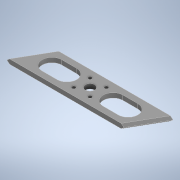
# Autodesk Inventor part: rotorV2
Saved by Autodesk Inventor 2021 (Build 250183000, 183)
## iProperties
Created: 2022-10-22
Part Number: rotorV2
Material: Generic
Document SubType Name: Modeling
Designer: ermoz
Density: 1 g/cm^3
Appearance: Default
Author: ermoz
Autodesk Inventor part; units mm, degrees
ref_plane "YZ Plane" through (0, 0, 0) normal (1, 0, 0) x (0, 1, 0)
ref_plane "XZ Plane" through (0, 0, 0) normal (0, 1, 0) x (-1, 0, 0)
ref_plane "XY Plane" through (0, 0, 0) normal (0, 0, 1) x (1, 0, 0)
sketch "Sketch1" plane through (0, 0, 0) normal (0, 1, 0) x (-1, 0, 0)
  circle A0 centre (0, 0) radius 13.5
  circle A1 centre (0, 0) radius 60
  line L0 (-58.4615, -13.5) -> (58.4615, -13.5)
  line L1 (58.4615, -13.5) -> (58.4615, 13.5)
  line L2 (58.4615, 13.5) -> (-58.4615, 13.5)
  line L3 (-58.4615, 13.5) -> (-58.4615, -13.5)
  line L4 (-58.4615, -13.5) -> (58.4615, 13.5) construction
  line L5 (58.4615, -13.5) -> (-58.4615, 13.5) construction
  line L6 (-20, 0) -> (-33, 0) construction
  line L7 (-20, 8.5) -> (-33, 8.5)
  line L8 (-33, -8.5) -> (-20, -8.5)
  arc A2 (-20, -8.5) -> (-20, 8.5) centre (-20, 0) ccw
  arc A3 (-33, 8.5) -> (-33, -8.5) centre (-33, 0) ccw
  line L9 (-58.4615, -13.5) -> (-42.8731, 13.5)
  line L10 (-58.4615, -13.5) -> (-27.2846, -13.5) construction
  line L11 (33, 0) -> (20, 0) construction
  line L12 (33, 8.5) -> (20, 8.5)
  line L13 (20, -8.5) -> (33, -8.5)
  arc A4 (33, -8.5) -> (33, 8.5) centre (33, 0) ccw
  arc A5 (20, 8.5) -> (20, -8.5) centre (20, 0) ccw
  line L14 (58.4615, 13.5) -> (47.2814, -5.8645)
  line L15 (58.4615, 13.5) -> (80.8217, 13.5) construction
  line L16 (47.2814, -5.8645) -> (42.8731, -13.5)
  point P0 (0, 0)
  point P1 (-0.767, 13.4782)
  point P2 (-9.0908, 9.9804)
  point P3 (0, 0)
  point P4 (-26.5, 0)
  point P5 (26.5, 0)
  point P6 (45.9853, -13.5)
  point P7 (0, 13.5)
  point P8 (0, -13.5)
  point P9 (12.75, -4.4371)
  point P10 (12.75, 4.4371)
  point P11 (-12.75, 4.4371)
  point P12 (-12.75, -4.4371)
  dimension "d7" = 120
  dimension "d1" = 27
  dimension "d9" = 5
  dimension "d10" = 5
  dimension "d11" = 60
  dimension "d12" = 5
  dimension "d13" = 5
  dimension "d14" = 13
  dimension "d15" = 13
  dimension "d16" = 20
  dimension "d17" = 20
  dimension "d24" = 120
  constraints: 38 end point, 10 point on circle, 9 tangent, 5 centre point, 5 horizontal, 5 midpoint, 4 parallel, 4 point on line, 2 coincident, 2 equal length, 1 perpendicular, 3 other
  measures "d1" diameter of A0
  measures "d9" distance between parallel lines of L0 L8
  measures "d10" distance between parallel lines of L2 L7
  measures "d11" angle of L10 L9
  measures "d12" distance between parallel lines of L0 L13
  measures "d13" distance between parallel lines of L2 L12
  measures "d14" distance of L6.end L6.start
  measures "d15" distance of L11.end L11.start
  measures "d16" distance of L6.start point (0, 0)
  measures "d17" distance of point (0, 0) L11.end
  measures "d24" angle of L14 L15
extrude "Extrusion1" add sketch "Sketch1" along normal blind 4 contours A5 A0 A2 | A0 L2 L14 L16 L0 A5 L13 A4 L12 | A0 A2 L7 A3 L8 L0 L9 L2
chamfer "Chamfer1" distance 2 angle 45 4 edges at (50.6673, 4, 0) (50.6673, 0, 0) (-52.8715, 0, 3.8177) (-52.8715, 4, 3.8177)
sketch "Sketch2" plane through (0, 4, 0) normal (0, 1, 0) x (1, 0, 0)
  circle A0 centre (0, 0) radius 4
  line L0 (0, 0) -> (7.0711, -7.0711)
  line L1 (0, 0) -> (10, 0) construction
  circle A1 centre (7.0711, -7.0711) radius 1.5
  circle A2 centre (7.0711, 7.0711) radius 1.5
  circle A3 centre (-7.0711, 7.0711) radius 1.5
  circle A4 centre (-7.0711, -7.0711) radius 1.5
  dimension "d21" = 8
  dimension "d31" = 10
  dimension "d32" = 45
  dimension "d33" = 3
  dimension "d36" = 360
  constraints: 5 centre point, 4 end point, 2 coincident, 1 equal length, 1 horizontal, 9 other
  measures "d21" diameter of A0
  measures "d31" distance of L0.start L0.end
  measures "d32" angle of L0 L1
  measures "d33" diameter of A1
extrude "Extrusion2" cut sketch "Sketch2" against normal blind 4
equation "\"d10\" = d9"
equation "\"d12\" = d9"
equation "\"d13\" = d9"
equation "\"d15\" = d14"
equation "\"d17\" = d16"
body "Solid1"
